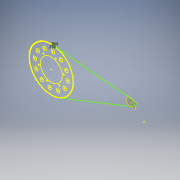
# Autodesk Inventor part: cadena2
Saved by Autodesk Inventor 2019.3 (Build 233278000, 278)
## iProperties
Created: 2018-12-14
Part Number: cadena2
Material: Generic
Document SubType Name: Modeling
Designer: eroldan
Density: 1 g/cm^3
Appearance: Default
Author: eroldan
Autodesk Inventor part; units mm, degrees
ref_plane "YZ Plane" through (0, 0, 0) normal (1, 0, 0) x (0, 1, 0)
ref_plane "XZ Plane" through (0, 0, 0) normal (0, 1, 0) x (-1, 0, 0)
ref_plane "XY Plane" through (0, 0, 0) normal (0, 0, 1) x (1, 0, 0)
ref_plane "Work Plane1" through (-50.9507, 50.6889, 57.5) normal (0, 0, 1) x (-0.2048689, -0.9787894, 0)
sketch "Sketch1" plane through (-50.9507, 50.6889, 57.5) normal (0, 0, 1) x (-0.2048689, -0.9787894, 0)
  arc A0 (13.9049, -7.4915) -> (-16.5454, -18.513) centre (0, -16.65) ccw
  circle A1 centre (79.9079, -408.7425) radius 3.175 projected
  circle A2 centre (121.7651, -356.8432) radius 3.175 projected
  circle A3 centre (187.6397, -367.1429) radius 3.175 projected
  circle A4 centre (211.6572, -429.3419) radius 3.175 projected
  circle A5 centre (169.8001, -481.2412) radius 3.175 projected
  circle A6 centre (103.9254, -470.9415) radius 3.175 projected
  circle A7 centre (66.2341, -383.8137) radius 9.5 projected
  circle A8 centre (136.5171, -332.537) radius 9.5 projected
  circle A9 centre (216.0656, -367.7655) radius 9.5 projected
  circle A10 centre (225.331, -454.2707) radius 9.5 projected
  circle A11 centre (155.048, -505.5474) radius 9.5 projected
  circle A12 centre (75.4996, -470.3189) radius 9.5 projected
  circle A13 centre (59.2774, -428.3076) radius 9.5 projected
  circle A14 centre (110.5541, -498.5906) radius 9.5 projected
  circle A15 centre (197.0593, -489.3252) radius 9.5 projected
  circle A16 centre (232.2878, -409.7768) radius 9.5 projected
  circle A17 centre (181.0111, -339.4938) radius 9.5 projected
  circle A18 centre (94.5059, -348.7592) radius 9.5 projected
  circle A19 centre (145.7826, -419.0422) radius 58 projected
  arc A20 (29.4913, -426.0124) -> (29.2993, -421.0163) centre (29.3729, -423.5152) ccw projected
  arc A21 (29.4913, -426.0124) -> (29.7056, -428.9608) centre (145.7826, -419.0422) ccw projected
  arc A22 (30.238, -433.9322) -> (29.7056, -428.9608) centre (29.9496, -431.4489) ccw projected
  arc A23 (30.238, -433.9322) -> (30.653, -436.8591) centre (145.7826, -419.0422) ccw projected
  arc A24 (31.5235, -441.7825) -> (30.653, -436.8591) centre (31.0663, -439.3247) ccw projected
  arc A25 (31.5235, -441.7825) -> (32.1373, -444.6743) centre (145.7826, -419.0422) ccw projected
  arc A26 (33.3417, -449.5268) -> (32.1373, -444.6743) centre (32.7178, -447.1059) ccw projected
  arc A27 (33.3417, -449.5268) -> (34.1514, -452.3699) centre (145.7826, -419.0422) ccw projected
  arc A28 (35.6842, -457.129) -> (34.1514, -452.3699) centre (34.8965, -454.7563) ccw projected
  arc A29 (35.6842, -457.129) -> (36.686, -459.9102) centre (145.7826, -419.0422) ccw projected
  arc A30 (38.54, -464.5536) -> (36.686, -459.9102) centre (37.5922, -462.2402) ccw projected
  arc A31 (38.54, -464.5536) -> (39.7293, -467.26) centre (145.7826, -419.0422) ccw projected
  arc A32 (41.8958, -471.766) -> (39.7293, -467.26) centre (40.7924, -469.5227) ccw projected
  arc A33 (41.8958, -471.766) -> (43.267, -474.3849) centre (145.7826, -419.0422) ccw projected
  arc A34 (45.736, -478.7325) -> (43.267, -474.3849) centre (44.4821, -476.5698) ccw projected
  arc A35 (45.736, -478.7325) -> (47.2827, -481.2518) centre (145.7826, -419.0422) ccw projected
  arc A36 (50.0427, -485.4208) -> (47.2827, -481.2518) centre (48.644, -483.3486) ccw projected
  arc A37 (50.0427, -485.4208) -> (51.7577, -487.8286) centre (145.7826, -419.0422) ccw projected
  arc A38 (54.7957, -491.7996) -> (51.7577, -487.8286) centre (53.2589, -489.8277) ccw projected
  arc A39 (54.7957, -491.7996) -> (56.671, -494.0847) centre (145.7826, -419.0422) ccw projected
  arc A40 (59.9729, -497.8391) -> (56.671, -494.0847) centre (58.3052, -495.9767) ccw projected
  arc A41 (59.9729, -497.8391) -> (61.9999, -499.991) centre (145.7826, -419.0422) ccw projected
  arc A42 (65.5503, -503.5113) -> (61.9999, -499.991) centre (63.7593, -501.767) ccw projected
  arc A43 (65.5503, -503.5113) -> (67.7193, -505.5198) centre (145.7826, -419.0422) ccw projected
  arc A44 (71.5017, -508.7896) -> (67.7193, -505.5198) centre (69.5959, -507.1716) ccw projected
  arc A45 (71.5017, -508.7896) -> (73.8027, -510.6454) centre (145.7826, -419.0422) ccw projected
  arc A46 (77.7994, -513.6495) -> (73.8027, -510.6454) centre (75.7876, -512.1654) ccw projected
  arc A47 (77.7994, -513.6495) -> (80.2218, -515.344) centre (145.7826, -419.0422) ccw projected
  arc A48 (84.4141, -518.0683) -> (80.2218, -515.344) centre (82.3058, -516.7249) ccw projected
  arc A49 (84.4141, -518.0683) -> (86.9465, -519.5935) centre (145.7826, -419.0422) ccw projected
  arc A50 (91.315, -522.0254) -> (86.9465, -519.5935) centre (89.1198, -520.829) ccw projected
  arc A51 (91.315, -522.0254) -> (93.9455, -523.3742) centre (145.7826, -419.0422) ccw projected
  arc A52 (98.4698, -525.5023) -> (93.9455, -523.3742) centre (96.1981, -524.4585) ccw projected
  arc A53 (98.4698, -525.5023) -> (101.1862, -526.6685) centre (145.7826, -419.0422) ccw projected
  arc A54 (105.8452, -528.4828) -> (101.1862, -526.6685) centre (103.5076, -527.5965) ccw projected
  arc A55 (105.8452, -528.4828) -> (108.6348, -529.4609) centre (145.7826, -419.0422) ccw projected
  arc A56 (113.4068, -530.9531) -> (108.6348, -529.4609) centre (111.0141, -530.2284) ccw projected
  arc A57 (113.4068, -530.9531) -> (116.2567, -531.7386) centre (145.7826, -419.0422) ccw projected
  arc A58 (121.1193, -532.9016) -> (116.2567, -531.7386) centre (118.6828, -532.3419) ccw projected
  arc A59 (121.1193, -532.9016) -> (124.0162, -533.4908) centre (145.7826, -419.0422) ccw projected
  arc A60 (128.9469, -534.3193) -> (124.0162, -533.4908) centre (126.4778, -533.9271) ccw projected
  arc A61 (128.9469, -534.3193) -> (131.8772, -534.7093) centre (145.7826, -419.0422) ccw projected
  arc A62 (136.8529, -535.1995) -> (131.8772, -534.7093) centre (134.3628, -534.9767) ccw projected
  arc A63 (136.8529, -535.1995) -> (139.803, -535.3886) centre (145.7826, -419.0422) ccw projected
  arc A64 (144.8006, -535.5381) -> (139.803, -535.3886) centre (142.3011, -535.4857) ccw projected
  arc A65 (144.8006, -535.5381) -> (147.7567, -535.5255) centre (145.7826, -419.0422) ccw projected
  arc A66 (152.7528, -535.3335) -> (147.7567, -535.5255) centre (150.2556, -535.4518) ccw projected
  arc A67 (152.7528, -535.3335) -> (155.7012, -535.1192) centre (145.7826, -419.0422) ccw projected
  arc A68 (160.6726, -534.5867) -> (155.7012, -535.1192) centre (158.1893, -534.8752) ccw projected
  arc A69 (160.6726, -534.5867) -> (163.5995, -534.1717) centre (145.7826, -419.0422) ccw projected
  arc A70 (168.5229, -533.3012) -> (163.5995, -534.1717) centre (166.0651, -533.7585) ccw projected
  arc A71 (168.5229, -533.3012) -> (171.4146, -532.6875) centre (145.7826, -419.0422) ccw projected
  arc A72 (176.2672, -531.483) -> (171.4146, -532.6875) centre (173.8463, -532.107) ccw projected
  arc A73 (176.2672, -531.483) -> (179.1103, -530.6733) centre (145.7826, -419.0422) ccw projected
  arc A74 (183.8694, -529.1405) -> (179.1103, -530.6733) centre (181.4967, -529.9282) ccw projected
  arc A75 (183.8694, -529.1405) -> (186.6506, -528.1387) centre (145.7826, -419.0422) ccw projected
  arc A76 (191.2939, -526.2847) -> (186.6506, -528.1387) centre (188.9806, -527.2325) ccw projected
  arc A77 (191.2939, -526.2847) -> (194.0003, -525.0955) centre (145.7826, -419.0422) ccw projected
  arc A78 (198.5063, -522.9289) -> (194.0003, -525.0955) centre (196.263, -524.0324) ccw projected
  arc A79 (198.5063, -522.9289) -> (201.1253, -521.5577) centre (145.7826, -419.0422) ccw projected
  arc A80 (205.4729, -519.0888) -> (201.1253, -521.5577) centre (203.3101, -520.3427) ccw projected
  arc A81 (205.4729, -519.0888) -> (207.9921, -517.542) centre (145.7826, -419.0422) ccw projected
  arc A82 (212.1612, -514.7821) -> (207.9921, -517.542) centre (210.089, -516.1807) ccw projected
  arc A83 (212.1612, -514.7821) -> (214.569, -513.0671) centre (145.7826, -419.0422) ccw projected
  arc A84 (218.54, -510.0291) -> (214.569, -513.0671) centre (216.5681, -511.5658) ccw projected
  arc A85 (218.54, -510.0291) -> (220.8251, -508.1537) centre (145.7826, -419.0422) ccw projected
  arc A86 (224.5795, -504.8518) -> (220.8251, -508.1537) centre (222.7171, -506.5196) ccw projected
  arc A87 (224.5795, -504.8518) -> (226.7314, -502.8249) centre (145.7826, -419.0422) ccw projected
  arc A88 (230.2517, -499.2745) -> (226.7314, -502.8249) centre (228.5074, -501.0655) ccw projected
  arc A89 (230.2517, -499.2745) -> (232.2602, -497.1055) centre (145.7826, -419.0422) ccw projected
  arc A90 (235.53, -493.3231) -> (232.2602, -497.1055) centre (233.912, -495.2289) ccw projected
  arc A91 (235.53, -493.3231) -> (237.3858, -491.022) centre (145.7826, -419.0422) ccw projected
  arc A92 (240.3899, -487.0253) -> (237.3858, -491.022) centre (238.9057, -489.0371) ccw projected
  arc A93 (240.3899, -487.0253) -> (242.0843, -484.603) centre (145.7826, -419.0422) ccw projected
  arc A94 (244.8087, -480.4106) -> (242.0843, -484.603) centre (243.4653, -482.519) ccw projected
  arc A95 (244.8087, -480.4106) -> (246.3339, -477.8783) centre (145.7826, -419.0422) ccw projected
  arc A96 (248.7657, -473.5098) -> (246.3339, -477.8783) centre (247.5693, -475.7049) ccw projected
  arc A97 (248.7657, -473.5098) -> (250.1146, -470.8793) centre (145.7826, -419.0422) ccw projected
  arc A98 (252.2427, -466.355) -> (250.1146, -470.8793) centre (251.1989, -468.6266) ccw projected
  arc A99 (252.2427, -466.355) -> (253.4088, -463.6386) centre (145.7826, -419.0422) ccw projected
  arc A100 (255.2232, -458.9796) -> (253.4088, -463.6386) centre (254.3369, -461.3172) ccw projected
  arc A101 (255.2232, -458.9796) -> (256.2013, -456.1899) centre (145.7826, -419.0422) ccw projected
  arc A102 (257.6935, -451.418) -> (256.2013, -456.1899) centre (256.9688, -453.8106) ccw projected
  arc A103 (257.6935, -451.418) -> (258.4789, -448.5681) centre (145.7826, -419.0422) ccw projected
  arc A104 (259.642, -443.7054) -> (258.4789, -448.5681) centre (259.0822, -446.142) ccw projected
  arc A105 (259.642, -443.7054) -> (260.2311, -440.8086) centre (145.7826, -419.0422) ccw projected
  arc A106 (261.0597, -435.8779) -> (260.2311, -440.8086) centre (260.6675, -438.3469) ccw projected
  arc A107 (261.0597, -435.8779) -> (261.4497, -432.9476) centre (145.7826, -419.0422) ccw projected
  arc A108 (261.9398, -427.9719) -> (261.4497, -432.9476) centre (261.717, -430.4619) ccw projected
  arc A109 (261.9398, -427.9719) -> (262.129, -425.0218) centre (145.7826, -419.0422) ccw projected
  arc A110 (262.2784, -420.0242) -> (262.129, -425.0218) centre (262.2261, -422.5236) ccw projected
  arc A111 (262.2784, -420.0242) -> (262.2658, -417.0681) centre (145.7826, -419.0422) ccw projected
  arc A112 (262.0739, -412.0719) -> (262.2658, -417.0681) centre (262.1922, -414.5691) ccw projected
  arc A113 (262.0739, -412.0719) -> (261.8596, -409.1236) centre (145.7826, -419.0422) ccw projected
  arc A114 (261.3271, -404.1522) -> (261.8596, -409.1236) centre (261.6156, -406.6355) ccw projected
  arc A115 (261.3271, -404.1522) -> (260.9121, -401.2253) centre (145.7826, -419.0422) ccw projected
  arc A116 (260.0416, -396.3019) -> (260.9121, -401.2253) centre (260.4989, -398.7597) ccw projected
  arc A117 (260.0416, -396.3019) -> (259.4278, -393.4101) centre (145.7826, -419.0422) ccw projected
  arc A118 (258.2234, -388.5576) -> (259.4278, -393.4101) centre (258.8473, -390.9785) ccw projected
  arc A119 (258.2234, -388.5576) -> (257.4137, -385.7145) centre (145.7826, -419.0422) ccw projected
  arc A120 (255.8809, -380.9554) -> (257.4137, -385.7145) centre (256.6686, -383.3281) ccw projected
  arc A121 (255.8809, -380.9554) -> (254.8791, -378.1742) centre (145.7826, -419.0422) ccw projected
  arc A122 (253.0251, -373.5308) -> (254.8791, -378.1742) centre (253.9729, -375.8442) ccw projected
  arc A123 (253.0251, -373.5308) -> (251.8358, -370.8244) centre (145.7826, -419.0422) ccw projected
  arc A124 (249.6693, -366.3184) -> (251.8358, -370.8244) centre (250.7727, -368.5617) ccw projected
  arc A125 (249.6693, -366.3184) -> (248.2981, -363.6995) centre (145.7826, -419.0422) ccw projected
  arc A126 (245.8291, -359.3519) -> (248.2981, -363.6995) centre (247.0831, -361.5146) ccw projected
  arc A127 (245.8291, -359.3519) -> (244.2824, -356.8326) centre (145.7826, -419.0422) ccw projected
  arc A128 (241.5225, -352.6636) -> (244.2824, -356.8326) centre (242.9211, -354.7358) ccw projected
  arc A129 (241.5225, -352.6636) -> (239.8075, -350.2558) centre (145.7826, -419.0422) ccw projected
  arc A130 (236.7695, -346.2848) -> (239.8075, -350.2558) centre (238.3062, -348.2567) ccw projected
  arc A131 (236.7695, -346.2848) -> (234.8941, -343.9996) centre (145.7826, -419.0422) ccw projected
  arc A132 (231.5922, -340.2453) -> (234.8941, -343.9996) centre (233.26, -342.1077) ccw projected
  arc A133 (231.5922, -340.2453) -> (229.5653, -338.0934) centre (145.7826, -419.0422) ccw projected
  arc A134 (226.0149, -334.5731) -> (229.5653, -338.0934) centre (227.8058, -336.3174) ccw projected
  arc A135 (226.0149, -334.5731) -> (223.8458, -332.5646) centre (145.7826, -419.0422) ccw projected
  arc A136 (220.0635, -329.2948) -> (223.8458, -332.5646) centre (221.9693, -330.9127) ccw projected
  arc A137 (220.0635, -329.2948) -> (217.7624, -327.439) centre (145.7826, -419.0422) ccw projected
  arc A138 (213.7657, -324.4349) -> (217.7624, -327.439) centre (215.7775, -325.919) ccw projected
  arc A139 (213.7657, -324.4349) -> (211.3434, -322.7404) centre (145.7826, -419.0422) ccw projected
  arc A140 (207.151, -320.0161) -> (211.3434, -322.7404) centre (209.2594, -321.3595) ccw projected
  arc A141 (207.151, -320.0161) -> (204.6187, -318.4909) centre (145.7826, -419.0422) ccw projected
  arc A142 (200.2501, -316.059) -> (204.6187, -318.4909) centre (202.4453, -317.2554) ccw projected
  arc A143 (200.2501, -316.059) -> (197.6196, -314.7102) centre (145.7826, -419.0422) ccw projected
  arc A144 (193.0953, -312.5821) -> (197.6196, -314.7102) centre (195.367, -313.6259) ccw projected
  arc A145 (193.0953, -312.5821) -> (190.3789, -311.4159) centre (145.7826, -419.0422) ccw projected
  arc A146 (185.72, -309.6015) -> (190.3789, -311.4159) centre (188.0576, -310.4879) ccw projected
  arc A147 (185.72, -309.6015) -> (182.9303, -308.6235) centre (145.7826, -419.0422) ccw projected
  arc A148 (178.1584, -307.1313) -> (182.9303, -308.6235) centre (180.551, -307.856) ccw projected
  arc A149 (178.1584, -307.1313) -> (175.3085, -306.3458) centre (145.7826, -419.0422) ccw projected
  arc A150 (170.4458, -305.1827) -> (175.3085, -306.3458) centre (172.8823, -305.7425) ccw projected
  arc A151 (170.4458, -305.1827) -> (167.5489, -304.5936) centre (145.7826, -419.0422) ccw projected
  arc A152 (162.6183, -303.7651) -> (167.5489, -304.5936) centre (165.0873, -304.1573) ccw projected
  arc A153 (162.6183, -303.7651) -> (159.688, -303.375) centre (145.7826, -419.0422) ccw projected
  arc A154 (154.7122, -302.8849) -> (159.688, -303.375) centre (157.2023, -303.1077) ccw projected
  arc A155 (154.7122, -302.8849) -> (151.7621, -302.6958) centre (145.7826, -419.0422) ccw projected
  arc A156 (146.7646, -302.5463) -> (151.7621, -302.6958) centre (149.264, -302.5987) ccw projected
  arc A157 (146.7646, -302.5463) -> (143.8084, -302.5589) centre (145.7826, -419.0422) ccw projected
  arc A158 (138.8123, -302.7509) -> (143.8084, -302.5589) centre (141.3095, -302.6326) ccw projected
  arc A159 (138.8123, -302.7509) -> (135.8639, -302.9652) centre (145.7826, -419.0422) ccw projected
  arc A160 (130.8926, -303.4977) -> (135.8639, -302.9652) centre (133.3759, -303.2092) ccw projected
  arc A161 (130.8926, -303.4977) -> (127.9657, -303.9127) centre (145.7826, -419.0422) ccw projected
  arc A162 (123.0422, -304.7832) -> (127.9657, -303.9127) centre (125.5001, -304.3259) ccw projected
  arc A163 (123.0422, -304.7832) -> (120.1505, -305.3969) centre (145.7826, -419.0422) ccw projected
  arc A164 (115.2979, -306.6014) -> (120.1505, -305.3969) centre (117.7188, -305.9774) ccw projected
  arc A165 (115.2979, -306.6014) -> (112.4548, -307.4111) centre (145.7826, -419.0422) ccw projected
  arc A166 (107.6958, -308.9438) -> (112.4548, -307.4111) centre (110.0684, -308.1562) ccw projected
  arc A167 (107.6958, -308.9438) -> (104.9145, -309.9457) centre (145.7826, -419.0422) ccw projected
  arc A168 (100.2712, -311.7996) -> (104.9145, -309.9457) centre (102.5846, -310.8519) ccw projected
  arc A169 (100.2712, -311.7996) -> (97.5648, -312.9889) centre (145.7826, -419.0422) ccw projected
  arc A170 (93.0588, -315.1555) -> (97.5648, -312.9889) centre (95.3021, -314.052) ccw projected
  arc A171 (93.0588, -315.1555) -> (90.4399, -316.5266) centre (145.7826, -419.0422) ccw projected
  arc A172 (86.0922, -318.9956) -> (90.4399, -316.5266) centre (88.255, -317.7417) ccw projected
  arc A173 (86.0922, -318.9956) -> (83.573, -320.5424) centre (145.7826, -419.0422) ccw projected
  arc A174 (79.404, -323.3023) -> (83.573, -320.5424) centre (81.4761, -321.9037) ccw projected
  arc A175 (79.404, -323.3023) -> (76.9961, -325.0173) centre (145.7826, -419.0422) ccw projected
  arc A176 (73.0252, -328.0553) -> (76.9961, -325.0173) centre (74.9971, -326.5185) ccw projected
  arc A177 (73.0252, -328.0553) -> (70.74, -329.9307) centre (145.7826, -419.0422) ccw projected
  arc A178 (66.9856, -333.2326) -> (70.74, -329.9307) centre (68.8481, -331.5648) ccw projected
  arc A179 (66.9856, -333.2326) -> (64.8338, -335.2595) centre (145.7826, -419.0422) ccw projected
  arc A180 (61.3135, -338.8099) -> (64.8338, -335.2595) centre (63.0577, -337.0189) ccw projected
  arc A181 (61.3135, -338.8099) -> (59.305, -340.9789) centre (145.7826, -419.0422) ccw projected
  arc A182 (56.0351, -344.7613) -> (59.305, -340.9789) centre (57.6531, -342.8555) ccw projected
  arc A183 (56.0351, -344.7613) -> (54.1793, -347.0624) centre (145.7826, -419.0422) ccw projected
  arc A184 (51.1753, -351.0591) -> (54.1793, -347.0624) centre (52.6594, -349.0473) ccw projected
  arc A185 (51.1753, -351.0591) -> (49.4808, -353.4814) centre (145.7826, -419.0422) ccw projected
  arc A186 (46.7565, -357.6738) -> (49.4808, -353.4814) centre (48.0999, -355.5654) ccw projected
  arc A187 (46.7565, -357.6738) -> (45.2313, -360.2061) centre (145.7826, -419.0422) ccw projected
  arc A188 (42.7994, -364.5746) -> (45.2313, -360.2061) centre (43.9958, -362.3795) ccw projected
  arc A189 (42.7994, -364.5746) -> (41.4506, -367.2051) centre (145.7826, -419.0422) ccw projected
  arc A190 (39.3225, -371.7294) -> (41.4506, -367.2051) centre (40.3663, -369.4577) ccw projected
  arc A191 (39.3225, -371.7294) -> (38.1563, -374.4458) centre (145.7826, -419.0422) ccw projected
  arc A192 (36.3419, -379.1048) -> (38.1563, -374.4458) centre (37.2283, -376.7672) ccw projected
  arc A193 (36.3419, -379.1048) -> (35.3638, -381.8945) centre (145.7826, -419.0422) ccw projected
  arc A194 (33.8716, -386.6664) -> (35.3638, -381.8945) centre (34.5964, -384.2738) ccw projected
  arc A195 (33.8716, -386.6664) -> (33.0862, -389.5163) centre (145.7826, -419.0422) ccw projected
  arc A196 (31.9231, -394.3789) -> (33.0862, -389.5163) centre (32.4829, -391.9424) ccw projected
  arc A197 (31.9231, -394.3789) -> (31.334, -397.2758) centre (145.7826, -419.0422) ccw projected
  arc A198 (30.5055, -402.2065) -> (31.334, -397.2758) centre (30.8977, -399.7374) ccw projected
  arc A199 (30.5055, -402.2065) -> (30.1154, -405.1368) centre (145.7826, -419.0422) ccw projected
  arc A200 (29.6253, -410.1125) -> (30.1154, -405.1368) centre (29.8481, -407.6225) ccw projected
  arc A201 (29.6253, -410.1125) -> (29.4361, -413.0626) centre (145.7826, -419.0422) ccw projected
  arc A202 (29.2867, -418.0602) -> (29.4361, -413.0626) centre (29.3391, -415.5607) ccw projected
  arc A203 (29.2867, -418.0602) -> (29.2993, -421.0163) centre (145.7826, -419.0422) ccw projected
  line L0 (-16.5454, -18.513) -> (29.9496, -431.4489)
  line L1 (13.9049, -7.4915) -> (247.0831, -361.5146)
  point P0 (39.1755, 60.2546)
  constraints: 4 end point, 2 point on circle, 2 tangent, 1 centre point
ref_plane "Work Plane2" through (-479.3841, 109.765, 57.5) normal (-0.9955659, 0.0940665, 0) x (-0.0940665, -0.9955659, 0)
sketch "Sketch2" plane through (-479.3841, 109.765, 57.5) normal (-0.9955659, 0.0940665, 0) x (-0.0940665, -0.9955659, 0)
  line L0 (-0.5181, 3.0742) -> (5.4819, 3.0742)
  line L1 (5.4819, 3.0742) -> (5.4819, -6.9258)
  line L2 (5.4819, -6.9258) -> (-0.5181, -6.9258)
  line L3 (-0.5181, -6.9258) -> (-0.5181, 3.0742)
  point P0 (64.1843, -57.5)
  dimension "d2" = 10
  dimension "d3" = 6
  constraints: 8 end point, 2 parallel, 1 horizontal, 1 perpendicular
  measures "d2" distance of L2.end L0.start
  measures "d3" distance of L0.start L0.end
sweep "Sweep1" add profiles "Sketch2" path "Sketch1" path curves L0 A0 L1
body "Solid2"
